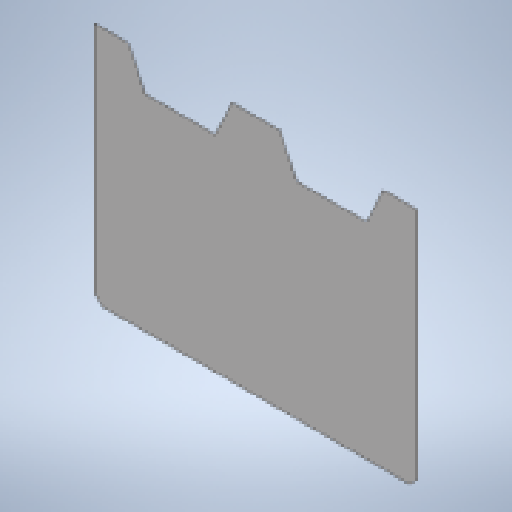
# Autodesk Inventor part: GBK-RK-0015 partition 5
Saved by Autodesk Inventor 2026.2 (Build 302298000, 298)
## iProperties
Created: 2026-09-14
Part Number: GBK-RK-0015 partition 5
Material: Generic
Document SubType Name: Sheet Metal
Designer: admin
Density: 1 g/cm^3
Sheet Metal Rule: Default_mm
Appearance: Default
Author: admin
Autodesk Inventor part; units mm, degrees
ref_plane "YZ Plane" through (0, 0, 0) normal (1, 0, 0) x (0, 1, 0)
ref_plane "XZ Plane" through (0, 0, 0) normal (0, 1, 0) x (-1, 0, 0)
ref_plane "XY Plane" through (0, 0, 0) normal (0, 0, 1) x (1, 0, 0)
sketch "Sketch3" plane through (0, 0, 0) normal (0, 0, 1) x (1, 0, 0)
  line L0 (735, 1100) -> (735, 35.3553)
  line L1 (735, 35.3553) -> (699.6447, 0)
  line L2 (699.6447, 0) -> (-699.6447, 0)
  line L3 (-699.6447, 0) -> (-735, 35.3553)
  line L4 (-735, 35.3553) -> (-735, 1100)
  line L5 (-735, 1100) -> (735, 1100)
  line L6 (0, 0) -> (0, 1100) construction
  line L7 (580.7856, 1100) -> (504.4788, 936.7568)
  line L8 (504.4788, 936.7568) -> (185.2514, 936.7568)
  line L9 (185.2514, 936.7568) -> (108.9446, 1100)
  line L10 (-108.9446, 1100) -> (-185.2514, 936.7568)
  line L11 (-185.2514, 936.7568) -> (-504.4788, 936.7568)
  line L12 (-504.4788, 936.7568) -> (-580.7856, 1100)
  dimension "d25" = 50
  dimension "d26" = 1100
  dimension "d27" = 1470
  measures "d25" distance of L2.end L3.end
  measures "d26" distance between parallel lines of L2 L5
  measures "d27" distance of L4.end L0.start
extrude "Plate3" add sketch "Sketch3" along normal blind 0.5 contours L0 L1 L2 L3 L4 L5 L12 L11 L10 L9 L8 L7
equation "\"d28\" = Thickness"
equation "\"BendRadius\" = Thickness"
equation "\"BendReliefWidth\" = Thickness"
equation "\"BendReliefDepth\" = 0.5 * Thickness"
equation "\"CornerReliefSize\" = 4 * Thickness"
equation "\"MinimumRemnant\" = 2 * Thickness"
equation "\"TransitionRadius\" = BendRadius"
equation "\"JacobiRadiusSize\" = BendRadius"
equation "\"GapSize\" = Thickness"
equation "\"Thickness\" = 0.5"
body "Solid2"
